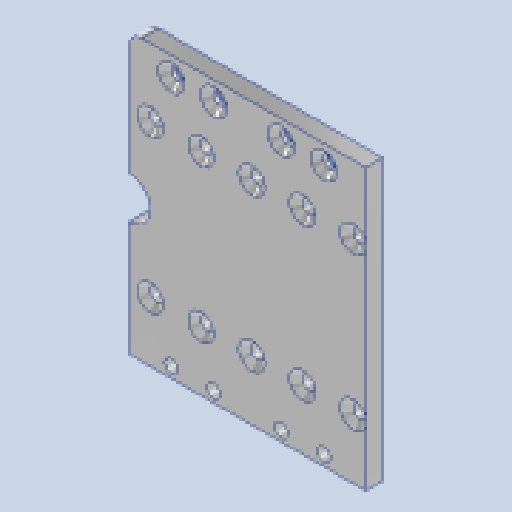
# Autodesk Inventor part: J1J2_Side
Saved by Autodesk Inventor 2023.1 (Build 271208000, 208)
## iProperties
Created: 2021-07-07
Part Number: J1J2_Side
Material: 알루미늄 6061
Document SubType Name: Modeling
Designer: user
Density: 2.7 g/cm^3
Appearance: 알루미늄 - 평지
Mass: 37.2871 g
Surface Area: 86.4597 cm^2
Volume: 13.81 cm^3
Author: user
Autodesk Inventor part; units mm, degrees
ref_plane "YZ Plane" through (0, 0, 0) normal (1, 0, 0) x (0, 1, 0)
ref_plane "XZ Plane" through (0, 0, 0) normal (0, 1, 0) x (-1, 0, 0)
ref_plane "XY Plane" through (0, 0, 0) normal (0, 0, 1) x (1, 0, 0)
sketch "스케치1" plane through (0, 0, 0) normal (0, 0, 1) x (1, 0, 0)
  line L0 (-28, 61.1) -> (28, 61.1)
  line L1 (28, 61.1) -> (28, -5.1)
  line L2 (28, -5.1) -> (-28, -5.1)
  line L3 (-28, -5.1) -> (-28, 61.1)
  point P0 (0, 0)
  dimension "d0" = 66.2
  dimension "d2" = 5.1
  dimension "d8" = 28
  dimension "d9" = 28
  constraints: 8 end point, 2 parallel, 1 horizontal, 1 perpendicular
  measures "d0" distance of L0.end L1.end
  measures "d2" distance from line of L2 point (0, 0)
  measures "d8" distance from line of L1 point (0, 0)
  measures "d9" distance from line of point (0, 0) L3
extrude "돌출1" add sketch "스케치1" along normal blind 4
sketch "스케치2" plane through (0, 0, 4) normal (0, 0, 1) x (1, 0, 0)
  line L0 (-2, 48) -> (-2, 6)
  line L1 (-32, 48) -> (-7.5, 48)
  line L2 (-2, 48) -> (4.5, 48)
  line L3 (16.5, 6) -> (16.5, 48)
  line L4 (10, 48) -> (16.5, 48)
  line L5 (10, 48) -> (10, 6)
  line L6 (10, 6) -> (16.5, 6)
  circle A0 centre (13, 45) radius 1.6
  circle A1 centre (13, 9) radius 1.6
  line L7 (28.5, 6) -> (28.5, 48)
  line L8 (22, 48) -> (28.5, 48)
  line L9 (22, 48) -> (22, 6)
  line L10 (22, 6) -> (28.5, 6)
  circle A2 centre (25, 45) radius 1.6
  circle A3 centre (25, 9) radius 1.6
  line L11 (-7.5, 6) -> (-7.5, 48)
  line L12 (-32, 48) -> (-7.5, 48)
  line L13 (-32, 48) -> (-32, 52)
  line L14 (-38, 52) -> (-32, 52)
  line L15 (-38, 2) -> (-38, 52)
  line L16 (-38, 2) -> (-32, 2)
  line L17 (-32, 2) -> (-32, 6)
  line L18 (-32, 6) -> (-7.5, 6)
  circle A4 centre (-35, 45) radius 1.6
  circle A5 centre (-35, 9) radius 1.6
  circle A6 centre (-23, 45) radius 1.6
  circle A7 centre (-23, 9) radius 1.6
  circle A8 centre (-11, 45) radius 1.6
  circle A9 centre (-11, 9) radius 1.6
  line L19 (-2, 6) -> (4.5, 6)
  circle A10 centre (1, 45) radius 1.6
  circle A11 centre (1, 9) radius 1.6
  line L20 (-2, 48) -> (0, 48)
  line L21 (0, 48) -> (0, 6)
  point P0 (0, 0)
  point P1 (-13, 26)
  dimension "d7" = 2
  constraints: 44 end point, 12 centre point, 2 point on line, 1 perpendicular
  measures "d7" distance of L0.start L20.end
extrude "돌출2" cut sketch "스케치2" against normal up to surface (4 mm away) contours L21 A10 | A10 L21 | L21 A11 | A11 L21 | A0 | A1 | A2 | A3 | A6 | A7 | A8 | A9
sketch "스케치3" plane through (0, 0, 4) normal (0, 0, 1) x (1, 0, 0)
  circle A0 centre (-23, 45) radius 1.6 projected
  circle A1 centre (-11, 45) radius 1.6 projected
  circle A2 centre (-11, 9) radius 1.6 projected
  circle A3 centre (25, 9) radius 1.6 projected
  circle A4 centre (13, 45) radius 1.6 projected
  circle A5 centre (1, 9) radius 1.6 projected
  circle A6 centre (1, 45) radius 1.6 projected
  circle A7 centre (13, 9) radius 1.6 projected
  circle A8 centre (25, 45) radius 1.6 projected
  circle A9 centre (-23, 9) radius 1.6 projected
  line L0 (28, 61.1) -> (-28, 61.1) projected
  line L1 (-28, 61.1) -> (-28, -5.1) projected
  line L2 (-28, -5.1) -> (28, -5.1) projected
  line L3 (28, -5.1) -> (28, 61.1) projected
  line L4 (-23, 45) -> (-23, 9)
  line L5 (-23, 27) -> (-28, 27)
  line L6 (-28, -5.1) -> (-28, 61.1) projected
  circle A10 centre (-28, 27) radius 5
  point P0 (0, 0)
  dimension "d12" = 18
  dimension "d15" = 10
  constraints: 4 end point, 1 centre point, 1 coincident, 1 horizontal, 1 midpoint, 1 point on line, 1 tangent, 1 vertical
  measures "d12" distance from line of L4.end L5
  measures "d15" diameter of A10
extrude "돌출3" cut sketch "스케치3" against normal blind 4 contours A10 L5 L1 | L1 A10 | L5 A10 L1
sketch "스케치4" plane through (0, 0, 4) normal (0, 0, 1) x (1, 0, 0)
  arc A0 (-28, 22) -> (-28, 32) centre (-28, 27) ccw projected
  line L0 (-28, 22) -> (-28, -5.1) projected
  line L1 (-28, -5.1) -> (28, -5.1) projected
  line L2 (28, -5.1) -> (28, 61.1) projected
  line L3 (28, 61.1) -> (-28, 61.1) projected
  line L4 (-28, 61.1) -> (-28, 32) projected
  circle A1 centre (-23, 9) radius 1.6 projected
  circle A2 centre (25, 45) radius 1.6 projected
  circle A3 centre (13, 9) radius 1.6 projected
  circle A4 centre (1, 45) radius 1.6 projected
  circle A5 centre (1, 9) radius 1.6 projected
  circle A6 centre (13, 45) radius 1.6 projected
  circle A7 centre (25, 9) radius 1.6 projected
  circle A8 centre (-11, 9) radius 1.6 projected
  circle A9 centre (-11, 45) radius 1.6 projected
  circle A10 centre (-23, 45) radius 1.6 projected
  circle A11 centre (-18, -2.6) radius 1.6
  circle A12 centre (-8, -2.6) radius 1.6
  circle A13 centre (8, -2.6) radius 1.6
  circle A14 centre (18, -2.6) radius 1.6
  point P0 (0, 0)
  dimension "d16" = 3.2
  dimension "d17" = 3.2
  dimension "d18" = 3.2
  dimension "d19" = 3.2
  dimension "d20" = 2.5
  dimension "d21" = 2.5
  dimension "d22" = 2.5
  dimension "d23" = 2.5
  dimension "d24" = 10
  dimension "d25" = 20
  dimension "d26" = 10
  dimension "d27" = 20
  constraints: 4 centre point
  measures "d16" diameter of A11
  measures "d17" diameter of A12
  measures "d18" diameter of A13
  measures "d19" diameter of A14
  measures "d20" distance from line of L1 A11.centre
  measures "d21" distance from line of L1 A12.centre
  measures "d22" distance from line of L1 A13.centre
  measures "d23" distance from line of L1 A14.centre
  measures "d24" distance from line of L0 A11.centre
  measures "d25" distance from line of L0 A12.centre
  measures "d26" distance from line of L2 A14.centre
  measures "d27" distance from line of L2 A13.centre
extrude "돌출4" cut sketch "스케치4" against normal up to surface (4 mm away) contours A11 | A12 | A13 | A14
sketch "스케치5" plane through (0, 0, 4) normal (0, 0, 1) x (1, 0, 0)
  circle A0 centre (8, -2.6) radius 1.6 projected
  circle A1 centre (18, -2.6) radius 1.6 projected
  circle A2 centre (-8, -2.6) radius 1.6 projected
  circle A3 centre (-18, -2.6) radius 1.6 projected
  arc A4 (-28, 22) -> (-28, 32) centre (-28, 27) ccw projected
  line L0 (-28, 22) -> (-28, -5.1) projected
  line L1 (-28, -5.1) -> (28, -5.1) projected
  line L2 (28, -5.1) -> (28, 61.1) projected
  line L3 (28, 61.1) -> (-28, 61.1) projected
  line L4 (-28, 61.1) -> (-28, 32) projected
  circle A5 centre (-23, 9) radius 1.6 projected
  circle A6 centre (25, 45) radius 1.6 projected
  circle A7 centre (13, 9) radius 1.6 projected
  circle A8 centre (1, 45) radius 1.6 projected
  circle A9 centre (1, 9) radius 1.6 projected
  circle A10 centre (13, 45) radius 1.6 projected
  circle A11 centre (25, 9) radius 1.6 projected
  circle A12 centre (-11, 9) radius 1.6 projected
  circle A13 centre (-11, 45) radius 1.6 projected
  circle A14 centre (-23, 45) radius 1.6 projected
  circle A15 centre (-18, 56.6) radius 1.6
  circle A16 centre (-8, 56.6) radius 1.6
  circle A17 centre (8, 56.6) radius 1.6
  circle A18 centre (18, 56.6) radius 1.6
  point P0 (0, 0)
  dimension "d30" = 3.2
  dimension "d31" = 3.2
  dimension "d32" = 3.2
  dimension "d33" = 3.2
  dimension "d34" = 4.5
  dimension "d35" = 4.5
  dimension "d36" = 4.5
  dimension "d37" = 4.5
  dimension "d38" = 10
  dimension "d39" = 20
  dimension "d40" = 10
  dimension "d41" = 20
  constraints: 4 centre point
  measures "d30" diameter of A15
  measures "d31" diameter of A16
  measures "d32" diameter of A17
  measures "d33" diameter of A18
  measures "d34" distance from line of L3 A15.centre
  measures "d35" distance from line of L3 A16.centre
  measures "d36" distance from line of L3 A17.centre
  measures "d37" distance from line of L3 A18.centre
  measures "d38" distance from line of L4 A15.centre
  measures "d39" distance from line of A16.centre L4
  measures "d40" distance from line of L2 A18.centre
  measures "d41" distance from line of L2 A17.centre
extrude "돌출5" cut sketch "스케치5" against normal up to surface (4 mm away) contours A15 | A16 | A17 | A18
fillet "모깎기1" radius 3 1 edges at (-28, 61.1, 2)
chamfer "모따기1" distance 1.5 angle 45 8 edges at (-19.6, 56.6, 4) (-9.6, 56.6, 4) (6.4, 56.6, 4) (16.4, 56.6, 4) (-19.6, 56.6, 0) (-9.6, 56.6, 0) (6.4, 56.6, 0) (16.4, 56.6, 0)
chamfer "모따기2" distance 1.5 angle 45 10 edges at (23.4, 45, 4) (11.4, 45, 4) (-0.6, 45, 4) (-12.6, 45, 4) (-24.6, 45, 4) (-24.6, 9, 4) (-12.6, 9, 4) (-0.6, 9, 4) (11.4, 9, 4) (23.4, 9, 4)
equation "\"d9\" = d8"
